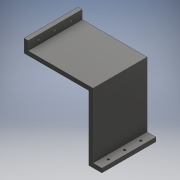
# Autodesk Inventor part: ConcreteFormwork2
Saved by Autodesk Inventor 2016 (Build 200138000, 138)
## iProperties
Created: 2015-06-07
Part Number: ConcreteFormwork2
Material: Wood (Birch)
Document SubType Name: Modeling
Designer: krosie
Density: 0.55 g/cm^3
Appearance: Birch - Natural Polished
Author: krosie
Autodesk Inventor part; units mm, degrees
ref_plane "YZ Plane" through (0, 0, 0) normal (1, 0, 0) x (0, 1, 0)
ref_plane "XZ Plane" through (0, 0, 0) normal (0, 1, 0) x (-1, 0, 0)
ref_plane "XY Plane" through (0, 0, 0) normal (0, 0, 1) x (1, 0, 0)
sketch "Sketch1" plane through (0, 0, 0) normal (0, 1, 0) x (-1, 0, 0)
  line L0 (300, 30) -> (300, -30)
  line L1 (300, -30) -> (0, -30)
  line L2 (0, -30) -> (0, -330)
  line L3 (0, -330) -> (-60, -330)
  point P0 (0, 0)
  dimension "d0" = 60
  dimension "d1" = 300
  dimension "d2" = 300
  dimension "d3" = 90
  dimension "d4" = 60
  dimension "d5" = 90
  constraints: 8 end point, 3 perpendicular, 1 vertical
  measures "d0" distance of L0.start L0.end
  measures "d1" distance of L0.end L1.end
  measures "d2" distance of L1.end L2.end
  measures "d3" angle of L2 L1
  measures "d4" distance of L2.end L3.end
  measures "d5" angle of L2 L3
surface extrude "ExtrusionSrf1" sketch "Sketch1" along normal blind 250 shown yes curves L0 L1 L2 L3
thicken "Thicken1" operation new thickness 19 both sides no extend neighbours no toward (1, 0, 0) faces at (-300, 166.6667, 10) (-200, 83.3333, -30) (0, 83.3333, -130) (20, 166.6667, -330)
hole "Hole1" at (-281, 200, 10) direction (-1, 0, 0) diameter 10 end through all
hole "Hole2" at (-281, 125, 10) direction (-1, 0, 0) diameter 10 end through all
hole "Hole3" at (-281, 50, 10) direction (-1, 0, 0) diameter 10 end through all
hole "Hole4" at (40, 200, -311) direction (0, 0, -1) diameter 10 end through all
hole "Hole5" at (40, 125, -311) direction (0, 0, -1) diameter 10 end through all
hole "Hole6" at (40, 50, -311) direction (0, 0, -1) diameter 10 end through all
body "Solid1"
body "Srf1"
